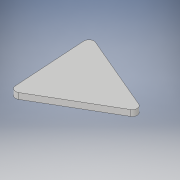
# Autodesk Inventor part: Vorfahrtsschild_Teil_Oben
Saved by Autodesk Inventor 2019.5 (Build 235369000, 369)
## iProperties
Created: 2021-10-06
Part Number: Vorfahrtsschild_Teil_Oben
Material: Generisch
Document SubType Name: Modeling
Designer: mritt
Density: 1 g/cm^3
Appearance: Vorgabe
Author: mritt
Autodesk Inventor part; units mm, degrees
ref_plane "YZ Plane" through (0, 0, 0) normal (1, 0, 0) x (0, 1, 0)
ref_plane "XZ Plane" through (0, 0, 0) normal (0, 1, 0) x (-1, 0, 0)
ref_plane "XY Plane" through (0, 0, 0) normal (0, 0, 1) x (1, 0, 0)
sketch "Skizze1" plane through (0, 0, 0) normal (0, 1, 0) x (-1, 0, 0)
  line L0 (71.8521, 103.64) -> (74.6911, 58.64)
  line L1 (74.6911, 58.64) -> (28.3832, 78.3082)
  line L2 (28.3832, 78.3082) -> (71.8521, 103.64)
  point P0 (0, 0)
  dimension "d16" = 45
  dimension "d17" = 50.3115
  dimension "d18" = 50.3115
  constraints: 6 end point
  measures "d16" vertical distance of L0.start L0.end
  measures "d17" distance of L1.end L0.start
  measures "d18" distance of L0.end L1.end
extrude "Extrusion2" add sketch "Skizze1" along normal blind 3
fillet "Rundung2" radius 2.5 3 edges at (-71.8521, 1.5, 103.64) (-74.6911, 1.5, 58.64) (-28.3832, 1.5, 78.3082)
